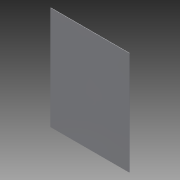
# Autodesk Inventor part: HeatSpreader
Saved by Autodesk Inventor 2015 (Build 190159000, 159)
## iProperties
Created: 2013-12-28
Part Number: HeatSpreader
Material: Aluminum 6061
Document SubType Name: Modeling
Designer: Jack
Density: 2.71 g/cm^3
Appearance: Aluminum - Flat
Author: Jack
Autodesk Inventor part; units mm, degrees
ref_plane "YZ Plane" through (0, 0, 0) normal (1, 0, 0) x (0, 1, 0)
ref_plane "XZ Plane" through (0, 0, 0) normal (0, 1, 0) x (-1, 0, 0)
ref_plane "XY Plane" through (0, 0, 0) normal (0, 0, 1) x (1, 0, 0)
sketch "Sketch1" plane through (0, 0, 0) normal (0, 1, 0) x (-1, 0, 0)
  line L0 (0, 0) -> (244, 0)
  line L1 (244, 0) -> (244, 314)
  line L2 (244, 314) -> (0, 314)
  line L3 (0, 314) -> (0, 0)
  dimension "d0" = 244
  dimension "d1" = 314
  constraints: 8 end point, 3 perpendicular, 1 horizontal
  measures "d0" distance of L0.start L0.end
  measures "d1" distance of L0.end L1.end
extrude "Extrusion1" add sketch "Sketch1" along normal blind 1.2
body "Solid1"
